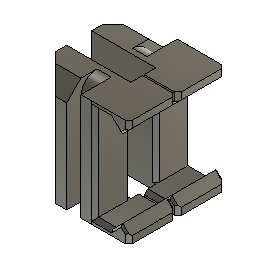
Compact_Robot_G3-G4 v6 (Autodesk Fusion 360 design; units mm, degrees)
Autodesk Fusion 360 part; units mm, degrees
sketch "Esboço1" plane through (0, 0, 0) normal (0, 0, 1) x (1, 0, 0)
  line L0 (0, 0) -> (-18, 0)
  line L1 (-18, 0) -> (-18, 3)
  line L2 (0, 0) -> (0, 10)
  line L3 (-18, 3) -> (-10.9996, 10.0004)
  line L4 (-10.9996, 10.0004) -> (0, 10)
  line L5 (-7.9996, 10.0003) -> (-3.9996, 10.0001)
  line L6 (-3.9996, 10.0001) -> (-3.9998, 6.0001)
  line L7 (-3.9998, 6.0001) -> (-7.9998, 6.0003)
  line L8 (-7.9998, 6.0003) -> (-7.9996, 10.0003)
  dimension "d1" = 18
  dimension "d2" = 3
  dimension "d3" = 10
  dimension "d5" = 135
  dimension "d6" = 9.9
  dimension "d10" = 4
  dimension "d11" = 4
  dimension "d12" = 4
  dimension "d13" = 4
  dimension "d14" = 3
  constraint coincident L0.start L2.start
  constraint horizontal L0
  constraint perpendicular L0 L1
  constraint perpendicular L0 L2
  constraint coincident L4 L5.start
  constraint parallel L4 L5
  constraint perpendicular L4 L6
  constraint perpendicular L6 L7
  constraint perpendicular L7 L8
  measures "d1" distance of L0.start L0.end
  measures "d2" distance of L0.end L1.end
  measures "d3" distance of L0.start L2.end
  measures "d5" angle of L1 L3
  measures "d6" distance of L1.end L3.end
  measures "d10" distance of L5.start L5.end
  measures "d11" distance of L5.end L6.end
  measures "d12" distance of L6.end L7.end
  measures "d13" distance of L7.end L5.start
  measures "d14" distance of L3.end L8
extrude "Extrusão1" add sketch "Esboço1" against normal blind 30 contours L0 L1 L2 L3 L4 L6 L7 L8 makes body 1
chamfer "Chanfro1" distance 4 angle 45 1 edges at (-9.4996, 10.0003, 0) on bodies 1
fillet "Arredondamento1" radius 4.5 2 edges at (-5.9998, 6.0002, 0) (-5.9998, 6.0002, -30) on bodies 1
sketch "Esboço2" plane through (0, 0, 0) normal (1, 0, 0) x (0, 1, 0)
  line L0 (10, 0) -> (0, 0)
  line L1 (0, 0) -> (0, -30)
  line L2 (0, -30) -> (10, -30)
  line L3 (10, -30) -> (10, 0)
  line L4 (10, 0) -> (-3.25, 0)
  line L5 (-3.25, 0) -> (-3.25, -1.75)
  line L6 (-3.25, -1.75) -> (10, -1.75)
  line L7 (10, -30) -> (-3.25, -30)
  line L8 (-3.25, -30) -> (-3.25, -28.25)
  line L9 (-3.25, -28.25) -> (10, -28.25)
  dimension "d20" = 13.25
  dimension "d21" = 1.75
  dimension "d22" = 13.25
  dimension "d23" = 1.75
  constraint coincident L0.start L3.end
  constraint perpendicular L3 L4
  constraint perpendicular L4 L5
  constraint coincident L3 L6.end
  constraint perpendicular L3 L6
  constraint coincident L2.end L3.start
  constraint perpendicular L1 L7
  constraint perpendicular L7 L8
  constraint coincident L3 L9.end
  constraint perpendicular L3 L9
  measures "d20" distance of L0.start L4.end
  measures "d21" distance of L4.end L5.end
  measures "d22" distance of L2.end L7.end
  measures "d23" distance of L7.end L8.end
extrude "Extrusão2" add sketch "Esboço2" along normal blind 9.4 contours L0 L1 L3 L4 L6 | L1 L4 L5 L6 | L1 L2 L3 L7 L9 | L1 L7 L8 L9 bodies 1
sketch "Esboço3" plane through (0, 10, 0) normal (0, 1, 0) x (-1, 0, 0)
  line L0 (0, -1.75) -> (0, 0)
  line L1 (0, 0) -> (-9.4, 0)
  line L2 (-9.4, 0) -> (-9.4, -1.75)
  line L3 (-9.4, -1.75) -> (0, -1.75)
  line L4 (-9.4, -1.75) -> (-9.4, -1.95)
  line L5 (0, -1.75) -> (0, -2.9)
  line L6 (-4.9, -1.75) -> (-7.2497, -4.0997)
  line L7 (-4.9, -1.75) -> (-4.75, -1.75)
  line L8 (-4.75, -1.75) -> (-4.75, -2.452)
  line L9 (-7.2497, -4.0997) -> (-9.5994, -1.75)
  dimension "d26" = 0.2
  dimension "d32" = 4.9
  dimension "d33" = 45
  dimension "d34" = 3.323
  dimension "d35" = 0.15
  dimension "d36" = 0.702
  dimension "d37" = 3.323
  constraint coincident L2.end L3.start
  constraint perpendicular L3 L4
  constraint coincident L0.start L3.end
  constraint perpendicular L3 L5
  constraint coincident L3 L6.start
  constraint parallel L3 L7
  constraint perpendicular L3 L8
  constraint perpendicular L6 L9
  measures "d26" distance of L2.end L4.end
  measures "d32" distance of L5 L6.start
  measures "d33" angle of L3 L6
  measures "d34" distance of L6.start L6.end
  measures "d35" distance of L6.start L7.end
  measures "d36" distance of L7.end L8.end
  measures "d37" distance of L6.end L9.end
sketch "Esboço4" plane through (0, 10, 0) normal (0, 1, 0) x (-1, 0, 0)
  line L0 (0, -30) -> (0, -28.25)
  line L1 (0, -28.25) -> (-9.4, -28.25)
  line L2 (-9.4, -28.25) -> (-9.4, -30)
  line L3 (-9.4, -30) -> (0, -30)
  line L4 (0, -28.25) -> (0, -26)
  line L5 (-9.4, -28.25) -> (-9.4, -28.05)
  line L6 (-4.9, -28.25) -> (-7.2497, -25.9003)
  line L7 (-7.2497, -25.9003) -> (-9.5994, -28.25)
  line L8 (-4.9, -28.25) -> (-4.75, -28.25)
  line L9 (-4.75, -28.25) -> (-4.75, -27.548)
  dimension "d38" = 0.2
  dimension "d39" = 3.323
  dimension "d40" = 4.9
  dimension "d41" = 45
  dimension "d42" = 3.323
  dimension "d43" = 0.15
  dimension "d44" = 0.702
  constraint coincident L0.end L1.start
  constraint perpendicular L1 L4
  constraint coincident L1.end L2.start
  constraint perpendicular L1 L5
  constraint coincident L1 L6.start
  constraint perpendicular L6 L7
  constraint parallel L1 L8
  constraint perpendicular L1 L9
  measures "d38" distance of L1.end L5.end
  measures "d39" distance of L6.start L6.end
  measures "d40" distance of L4 L6.start
  measures "d41" angle of L1 L6
  measures "d42" distance of L6.end L7.end
  measures "d43" distance of L6.start L8.end
  measures "d44" distance of L8.end L9.end
extrude "Extrusão3" add sketch "Esboço4" sketch "Esboço3" against normal blind 13.25 contours L1 L5 L6 L7 of sketch 2 contours L3 L4 L6 L9 bodies 1
chamfer "Chanfro2" distance 0.5 angle 45 8 edges at (6.0749, 10, -2.9249) (8.3249, 10, -3.0246) (6.0749, 10, -27.0751) (8.3249, 10, -26.9754) (8.3249, -3.25, -3.0246) (6.0749, -3.25, -2.9249) (8.3249, -3.25, -26.9754) (6.0749, -3.25, -27.0751) on bodies 1
chamfer "Chanfro3" distance 1 angle 45 8 edges at (9.4, -3.25, -0.6212) (2.8036, -3.25, -1.75) (2.8036, -3.25, -28.25) (9.4, -3.25, -29.3788) (9.4, 10, -29.3788) (2.8036, 10, -28.25) (9.4, 10, -0.6212) (2.8036, 10, -1.75) on bodies 1
chamfer "Chanfro4" distance 1 angle 45 2 edges at (0, 10, -15) (0, 0, -15) on bodies 1
ref_plane "Plano de trabalho1" through (0, -3.5, 0) normal (0, 1, 0) x (0, 0, 1)
mirror "Espelhar1" about plane through (0, -3.5, 0) normal (0, 1, 0) of bodies 1 makes body 2
